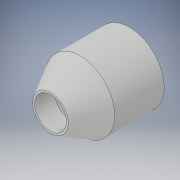
# Autodesk Inventor part: blocage_recule_support_douille
Saved by Autodesk Inventor 2019 (Build 230136000, 136)
## iProperties
Created: 2019-03-25
Part Number: blocage_recule_support_douille
Material: Générique
Document SubType Name: Modeling
Designer: theor
Density: 1 g/cm^3
Appearance: Par défaut
Author: theor
Autodesk Inventor part; units mm, degrees
ref_plane "YZ Plane" through (0, 0, 0) normal (1, 0, 0) x (0, 1, 0)
ref_plane "XZ Plane" through (0, 0, 0) normal (0, 1, 0) x (-1, 0, 0)
ref_plane "XY Plane" through (0, 0, 0) normal (0, 0, 1) x (1, 0, 0)
sketch "Esquisse1" plane through (0, 0, 0) normal (1, 0, 0) x (0, 1, 0)
  line L0 (0, 0) -> (0, 36.6667)
  line L1 (17.5, 0) -> (17.5, 25)
  line L2 (17.5, 0) -> (11, 0)
  line L3 (17.5, 25) -> (9, 40)
  line L4 (9, 40) -> (8, 40)
  line L5 (8, 40) -> (8, 30)
  line L6 (8, 30) -> (10, 30)
  line L7 (10, 30) -> (13, 25)
  line L8 (13, 25) -> (13, 3)
  line L9 (13, 3) -> (11, 3)
  line L10 (11, 0) -> (11, 3)
  dimension "d0" = 35
  dimension "d1" = 16
  dimension "d2" = 1
  dimension "d3" = 2
  dimension "d4" = 26
  dimension "d7" = 5
  dimension "d8" = 10
  dimension "d11" = 30
  dimension "d12" = 22
  dimension "d13" = 3
  constraints: 22 end point, 5 vertical, 4 horizontal, 2 horizontal alignment
  measures "d0" diameter of L1 L0
  measures "d1" diameter of L5 L0
  measures "d2" distance of L3.end L4.end
  measures "d3" distance of L5.end L6.end
  measures "d4" diameter of L7.end L0
  measures "d7" vertical distance of L6.end L7.end
  measures "d8" distance between parallel lines of L4 L6
  measures "d11" distance from line of L2.end L6
  measures "d12" diameter of L10 L0
  measures "d13" distance of L2.end L9.end
revolve "Révolution1" add sketch "Esquisse1" angle 360 about axis through (0, 0, 0) along (0, 0, 1)
